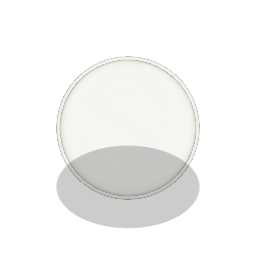
球 v1 (Autodesk Fusion 360 design; units mm, degrees)
Autodesk Fusion 360 part; units mm, degrees
sketch "スケッチ1" plane through (0, 0, 0) normal (1, 0, 0) x (0, 0, -1)
  arc A0 (0, 42) -> (0, -42) centre (0, 0) ccw
  arc A1 (0, 40) -> (0, -40) centre (0, 0) ccw
  line L0 (0, -42) -> (0, -40)
  line L1 (0, 40) -> (0, 42)
  dimension "d3" = 42
  dimension "d4" = 40
  measures "d3" radius of A0
  measures "d4" radius of A1
revolve "回転1" add sketch "スケッチ1" angle 360 about axis through (0, 1.75, 0) along (0, 1, 0)
